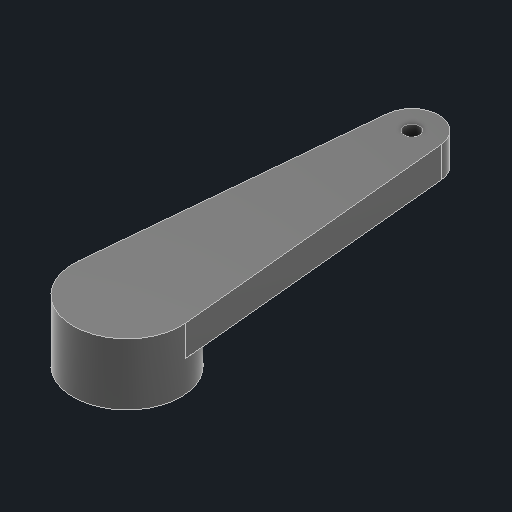
# Autodesk Inventor part: servohorn
Saved by Autodesk Inventor 2024 (Build 280153000, 153)
## iProperties
Created: 2025-01-02
Part Number: servohorn
Material: Acetal Resin, Black
Document SubType Name: Modeling
Designer: huj31
Density: 1.425 g/cm^3
Appearance: Smooth - Black
Author: huj31
Autodesk Inventor part; units mm, degrees
ref_plane "YZ Plane" through (0, 0, 0) normal (1, 0, 0) x (0, 1, 0)
ref_plane "XZ Plane" through (0, 0, 0) normal (0, 1, 0) x (-1, 0, 0)
ref_plane "XY Plane" through (0, 0, 0) normal (0, 0, 1) x (1, 0, 0)
sketch "Sketch1" plane through (0, 0, 0) normal (0, 1, 0) x (-1, 0, 0)
  circle A0 centre (0, 0) radius 3.5
  line L0 (0, 3.5) -> (0, -18.5)
  circle A1 centre (0, -18.5) radius 1.75
  line L1 (1.7422, -18.6655) -> (3.4843, -0.3311)
  line L2 (-1.7422, -18.6655) -> (-3.4843, -0.3311)
  circle A2 centre (0, 0) radius 2.5
  circle A3 centre (0, -18.5) radius 0.5
  dimension "d0" = 7
  dimension "d1" = 22
  dimension "d2" = 3.5
  dimension "d3" = 5
  dimension "d8" = 1
  constraints: 6 end point, 5 point on circle, 4 centre point, 4 coincident, 4 tangent, 2 vertical
  measures "d0" diameter of A0
  measures "d1" distance of L0.start L0.end
  measures "d2" diameter of A1
  measures "d3" diameter of A2
  measures "d8" diameter of A3
extrude "Extrusion1" add sketch "Sketch1" along normal blind 2
extrude "Extrusion2" add sketch "Sketch1" against normal blind 2 contours A0 L0 A2 | L0 A2 A0
body "Solid1"
